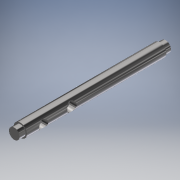
# Autodesk Inventor part: Mecanum Axle
Saved by Autodesk Inventor 2019.4 (Build 234330000, 330)
## iProperties
Created: 2019-10-19
Part Number: Mecanum Axle
Material: Stainless Steel
Document SubType Name: Modeling
Designer: admin
Density: 8 g/cm^3
Appearance: Semi-Polished
Author: admin
Autodesk Inventor part; units mm, degrees
ref_plane "YZ Plane" through (0, 0, 0) normal (1, 0, 0) x (0, 1, 0)
ref_plane "XZ Plane" through (0, 0, 0) normal (0, 1, 0) x (-1, 0, 0)
ref_plane "XY Plane" through (0, 0, 0) normal (0, 0, 1) x (1, 0, 0)
sketch "Sketch1" plane through (0, 0, 0) normal (1, 0, 0) x (0, 1, 0)
  line L0 (0, 0) -> (4, 0)
  line L1 (4, 0) -> (4, -4.5)
  line L2 (4, -4.5) -> (5, -4.5)
  line L3 (5, -4.5) -> (5, -109.3)
  line L4 (5, -109.3) -> (4, -109.3)
  line L5 (4, -109.3) -> (4, -113.8)
  line L6 (4, -113.8) -> (0, -113.8)
  line L7 (0, -113.8) -> (0, 0)
  dimension "d0" = 4.5
  dimension "d1" = 113.8
  dimension "d2" = 5
  dimension "d3" = 4
  dimension "d4" = 4
  dimension "d5" = 4.5
  constraints: 16 end point, 7 perpendicular, 1 horizontal
  measures "d0" distance of L0.end L1.end
  measures "d1" distance between parallel lines of L6 L0
  measures "d2" distance between parallel lines of L7 L3
  measures "d3" distance between parallel lines of L7 L1
  measures "d4" distance between parallel lines of L7 L5
  measures "d5" distance of L4.end L5.end
revolve "Revolution1" add sketch "Sketch1" angle 360 about axis through (0, 0, -113.8) along (0, 0, 1)
sketch "Sketch2" plane through (0, 0, 0) normal (1, 0, 0) x (0, 1, 0)
  circle A0 centre (-0.6781, -17.2) radius 3.5
  line L0 (-4, 0) -> (4, 0) projected
  point P0 (0, 0)
  dimension "d7" = 7
  dimension "d8" = 17.2
  constraints: 1 centre point
  measures "d7" diameter of A0
  measures "d8" distance from line of L0 A0.centre
extrude "Extrusion1" cut sketch "Sketch2" along normal through all
sketch "Sketch3" plane through (0, 0, 0) normal (1, 0, 0) x (0, 1, 0)
  circle A0 centre (0.378, -38.4) radius 3.5
  line L0 (-4, -113.8) -> (4, -113.8) projected
  point P0 (0, 0)
  dimension "d11" = 7
  dimension "d12" = 75.4
  constraints: 1 centre point
  measures "d11" diameter of A0
  measures "d12" distance from line of L0 A0.centre
extrude "Extrusion2" cut sketch "Sketch3" along normal through all
equation "\"d5\" = d0"
body "Solid1"
